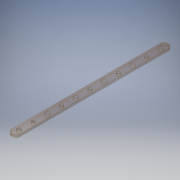
# Autodesk Inventor part: Bearing Holder
Saved by Autodesk Inventor 2019.4 (Build 234330000, 330)
## iProperties
Created: 2020-01-11
Part Number: Bearing Holder
Material: Polycarbonate, Smoke
Document SubType Name: Modeling
Designer: admin
Density: 1.2 g/cm^3
Appearance: Polycarbonate - Smoked
Mass: 6.95374 g
Surface Area: 54.4277 cm^2
Volume: 5.79479 cm^3
Author: admin
Autodesk Inventor part; units mm, degrees
ref_plane "YZ Plane" through (0, 0, 0) normal (1, 0, 0) x (0, 1, 0)
ref_plane "XZ Plane" through (0, 0, 0) normal (0, 1, 0) x (-1, 0, 0)
ref_plane "XY Plane" through (0, 0, 0) normal (0, 0, 1) x (1, 0, 0)
sketch "Sketch1" plane through (0, 0, 0) normal (0, 1, 0) x (-1, 0, 0)
  line L0 (-6, 110) -> (6, 110)
  line L1 (6, 110) -> (6, -110)
  line L2 (6, -110) -> (-6, -110)
  line L3 (-6, -110) -> (-6, 110)
  line L4 (-6, 110) -> (6, -110) construction
  line L5 (6, 110) -> (-6, -110) construction
  line L6 (0, 100) -> (0, -100) construction
  circle A0 centre (0, 100) radius 3.05
  circle A1 centre (0, 60) radius 3.05
  circle A2 centre (0, -60) radius 3.05
  circle A3 centre (0, -100) radius 3.05
  circle A4 centre (0, 80) radius 2.2
  circle A5 centre (0, 40) radius 2.2
  circle A6 centre (0, 0) radius 2.2
  circle A7 centre (0, -40) radius 2.2
  circle A8 centre (0, 20) radius 3.05
  circle A9 centre (0, -20) radius 3.05
  circle A10 centre (0, -80) radius 2.2
  dimension "d0" = 6.1
  dimension "d1" = 6.1
  dimension "d2" = 6.1
  dimension "d3" = 6.1
  dimension "d4" = 40
  dimension "d6" = 40
  dimension "d7" = 10
  dimension "d10" = 12
  dimension "d11" = 4.4
  dimension "d12" = 4.4
  dimension "d13" = 4.4
  dimension "d14" = 4.4
  dimension "d15" = 40
  dimension "d16" = 40
  dimension "d17" = 40
  dimension "d18" = 20
  dimension "d22" = 6.1
  dimension "d23" = 6.1
  dimension "d24" = 4.4
  dimension "d25" = 40
  dimension "d26" = 40
  dimension "d27" = 40
  constraints: 12 end point, 11 centre point, 4 midpoint, 2 coincident, 2 parallel, 1 horizontal, 1 perpendicular, 13 other
  measures "d0" diameter of A0
  measures "d1" diameter of A1
  measures "d2" diameter of A2
  measures "d3" diameter of A3
  measures "d4" distance of A1.centre A0.centre
  measures "d6" distance of A3.centre A2.centre
  measures "d7" distance from line of L2 A3.centre
  measures "d10" distance of L1.end L2.end
  measures "d11" diameter of A4
  measures "d12" diameter of A5
  measures "d13" diameter of A6
  measures "d14" diameter of A7
  measures "d15" distance of A5.centre A4.centre
  measures "d16" distance of A6.centre A5.centre
  measures "d17" distance of A6.centre A7.centre
  measures "d18" distance of A0.centre A4.centre
  measures "d22" diameter of A8
  measures "d23" diameter of A9
  measures "d24" diameter of A10
  measures "d25" distance of A1.centre A8.centre
  measures "d26" distance of A9.centre A8.centre
  measures "d27" distance of A10.centre A7.centre
extrude "Extrusion1" add sketch "Sketch1" along normal blind 3
fillet "Fillet1" radius 5 4 edges at (-6, 1.5, 110) (6, 1.5, 110) (-6, 1.5, -110) (6, 1.5, -110)
equation "\"d18\" = 0.5 * d4"
body "Solid1"
